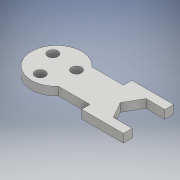
# Autodesk Inventor part: Деталь1 Курганова
Saved by Autodesk Inventor 2017 (Build 210142000, 142)
## iProperties
Part Number: Деталь1 Курганова
Material: Типовые
Document SubType Name: Modeling
Designer: Sasha
Density: 1 g/cm^3
Appearance: По умолчанию
Mass: 7.1013 g
Surface Area: 42.5122 cm^2
Volume: 7.1013 cm^3
Author: Sasha
Autodesk Inventor part; units mm, degrees
ref_plane "YZ Plane" through (0, 0, 0) normal (1, 0, 0) x (0, 1, 0)
ref_plane "XZ Plane" through (0, 0, 0) normal (0, 1, 0) x (-1, 0, 0)
ref_plane "XY Plane" through (0, 0, 0) normal (0, 0, 1) x (1, 0, 0)
sketch "Эскиз1" plane through (0, 0, 0) normal (0, 0, 1) x (1, 0, 0)
  arc A0 (11.1803, 10) -> (11.1803, -10) centre (0, 0) ccw
  line L0 (30, 15) -> (55, 15)
  line L1 (55, -15) -> (30, -15)
  line L2 (30, -15) -> (30, 15)
  line L3 (11.1803, 10) -> (30, 10)
  line L4 (11.1803, -10) -> (30, -10)
  line L5 (-7.3724, 5.1622) -> (0, 0)
  line L6 (0, 9) -> (0, 0)
  circle A1 centre (-7.3724, 5.1622) radius 3
  circle A2 centre (-0.7844, -8.9658) radius 3
  circle A3 centre (8.1568, 3.8036) radius 3
  line L7 (55, -9.7741) -> (43.7138, -9.7741)
  line L8 (43.7138, -9.7741) -> (38.0707, 0)
  line L9 (38.0707, 0) -> (43.7138, 9.7741)
  line L10 (43.7138, 9.7741) -> (55, 9.7741)
  line L11 (55, 9.7741) -> (54.9588, 9.8455)
  line L12 (55, 15) -> (55, 9.7741)
  line L13 (55, -9.7741) -> (55, -15)
  point P0 (49.3569, 0)
  dimension "d0" = 15
  dimension "d1" = 25
  dimension "d2" = 30
  dimension "d3" = 15
  dimension "d4" = 30
  dimension "d5" = 10
  dimension "d6" = 20
  dimension "d8" = 9
  dimension "d9" = 55
  dimension "d10" = 6
  dimension "d13" = 360
  constraints: 29 end point, 4 centre point, 4 horizontal, 3 parallel, 2 coincident, 2 equal length, 2 perpendicular, 2 point on circle, 2 point on line, 1 horizontal alignment, 1 vertical, 16 other
  measures "d0" radius of A0
  measures "d1" distance of L0.start L0.end
  measures "d2" distance of L0.end L1.start
  measures "d3" distance from line of L5.end L0
  measures "d4" distance from line of L2 L5.end
  measures "d5" distance from line of L5.end L3
  measures "d6" distance between parallel lines of L4 L3
  measures "d8" distance of L6.start L5.end
  measures "d9" angle of L6 L5
  measures "d10" diameter of A1
extrude "Выдавливание1" add sketch "Эскиз1" along normal blind 5
